Autodesk Fusion 360 part; units mm, degrees
note: some values were not read from the file. Chosen so that the rebuilt part matches the saved one: which bodies a step acts on; which face or edge a step refers to. Set by a fixed rule: which sketch regions a step uses.
(part 2 of 2)
chamfer "Chamfer1" distance 0.1 angle 45 2 edges at (2.2467, -480.7059, 0) (382.2081, -629.6946, 0) on bodies 3 in component "Side_Panel"
sketch "Sketch1 (2)" plane through (0, 0, 0) normal (0, 0, 1) x (-1, 0, 0) in component "Side_Panel"
  circle A0 centre (-385.0517, 697.8099) radius 3.15
  circle A1 centre (-364.1017, 475.8227) radius 3.15
  circle A2 centre (-226.7218, 475.8227) radius 3.15
  circle A3 centre (-108.0319, 475.8227) radius 3.15
  circle A4 centre (29.3479, 475.8227) radius 3.15
  circle A5 centre (118.9878, 496.7727) radius 3.15
  circle A6 centre (118.9878, 630.7975) radius 3.15
  circle A7 centre (118.9878, 697.8099) radius 3.15
  circle A8 centre (118.9878, 563.7851) radius 3.15
  circle A9 centre (98.0378, 475.8227) radius 3.15
  circle A10 centre (-39.342, 475.8227) radius 3.15
  circle A11 centre (-158.0319, 475.8227) radius 3.15
  circle A12 centre (-295.4117, 475.8227) radius 3.15
  circle A13 centre (-385.0517, 496.7727) radius 3.15
  circle A14 centre (-385.0517, 563.7851) radius 3.15
  arc A15 (-5.547, 484.7727) -> (-4.447, 484.7727) centre (-4.997, 481.7727) ccw
  line L0 (-5.547, 484.7727) -> (-82.4819, 484.7727)
  arc A16 (-83.5819, 484.7727) -> (-82.4819, 484.7727) centre (-83.0319, 481.7727) ccw
  line L1 (-83.5819, 484.7727) -> (-182.4819, 484.7727)
  arc A17 (-183.5819, 484.7727) -> (-182.4819, 484.7727) centre (-183.0319, 481.7727) ccw
  line L2 (-183.5819, 484.7727) -> (-260.5168, 484.7727)
  arc A18 (-261.6168, 484.7727) -> (-260.5168, 484.7727) centre (-261.0668, 481.7727) ccw
  line L3 (-261.6168, 484.7727) -> (-338.5517, 484.7727)
  arc A19 (-339.6517, 484.7727) -> (-338.5517, 484.7727) centre (-339.1017, 481.7727) ccw
  line L4 (-339.6517, 484.7727) -> (-376.1017, 484.7727)
  line L5 (-376.1017, 484.7727) -> (-376.1017, 521.2227)
  arc A20 (-376.1017, 522.3227) -> (-376.1017, 521.2227) centre (-379.1017, 521.7727) ccw
  line L6 (-376.1017, 522.3227) -> (-376.1017, 596.7413)
  arc A21 (-376.1017, 597.8413) -> (-376.1017, 596.7413) centre (-379.1017, 597.2913) ccw
  line L7 (-376.1017, 597.8413) -> (-376.1017, 672.2599)
  arc A22 (-376.1017, 673.3599) -> (-376.1017, 672.2599) centre (-379.1017, 672.8099) ccw
  line L8 (-376.1017, 673.3599) -> (-376.1017, 722.8099)
  line L9 (-376.1017, 722.8099) -> (-387.1017, 722.8099)
  line L10 (-387.1017, 722.8099) -> (-387.1017, 702.8099)
  arc A23 (-389.1017, 700.8099) -> (-387.1017, 702.8099) centre (-389.1017, 702.8099) ccw
  line L11 (-389.1017, 700.8099) -> (-389.1017, 473.7727)
  arc A24 (-389.1017, 473.7727) -> (-387.1017, 471.7727) centre (-387.1017, 473.7727) ccw
  line L12 (-387.1017, 471.7727) -> (-155.0319, 471.7727)
  arc A25 (-153.0319, 473.7727) -> (-155.0319, 471.7727) centre (-153.0319, 471.7727) ccw
  line L13 (-153.0319, 473.7727) -> (-113.0319, 473.7727)
  arc A26 (-111.0319, 471.7727) -> (-113.0319, 473.7727) centre (-113.0319, 471.7727) ccw
  line L14 (-111.0319, 471.7727) -> (121.0378, 471.7727)
  arc A27 (121.0378, 471.7727) -> (123.0378, 473.7727) centre (121.0378, 473.7727) ccw
  line L15 (123.0378, 473.7727) -> (123.0378, 700.8099)
  arc A28 (121.0378, 702.8099) -> (123.0378, 700.8099) centre (123.0378, 702.8099) ccw
  line L16 (121.0378, 702.8099) -> (121.0378, 722.8099)
  line L17 (121.0378, 722.8099) -> (110.0378, 722.8099)
  line L18 (110.0378, 722.8099) -> (110.0378, 673.3599)
  arc A29 (110.0378, 672.2599) -> (110.0378, 673.3599) centre (113.0378, 672.8099) ccw
  line L19 (110.0378, 672.2599) -> (110.0378, 597.8413)
  arc A30 (110.0378, 596.7413) -> (110.0378, 597.8413) centre (113.0378, 597.2913) ccw
  line L20 (110.0378, 596.7413) -> (110.0378, 522.3227)
  arc A31 (110.0378, 521.2227) -> (110.0378, 522.3227) centre (113.0378, 521.7727) ccw
  line L21 (110.0378, 521.2227) -> (110.0378, 484.7727)
  line L22 (110.0378, 484.7727) -> (73.5878, 484.7727)
  arc A32 (72.4878, 484.7727) -> (73.5878, 484.7727) centre (73.0378, 481.7727) ccw
  line L23 (72.4878, 484.7727) -> (-4.447, 484.7727)
  circle A33 centre (-385.0517, 630.7975) radius 3.15
  line L24 (-133.0319, 473.7727) -> (-133.0319, 484.7727)
  constraint midpoint L13 L24.start
  constraint midpoint L1 L24.end
split "Split1'" by curves path "Sketch1 (2)" along L24 bodies 3 makes body 4 at (-115.4304, -706.7068, -4) in component "Side_Panel"
chamfer "Chamfer2'" distance 0.4 angle 45 2 faces at (-115.4304, -706.7068, -4) (381.6101, -706.6822, -4) on bodies 3 4 in component "Side_Panel"
extrude "Extrude17" add sketch "Master Sketch" against normal blind 5 separate body contours L21 L24 L27 L28 A72 L41 L42 A150 | L22 A53 L24 L27 L28 L29 L32 A62 A63 L35 L36 A72 A150 | L21 L28 L39 L41 L42 | L27 A150 | L27 A150 | A53 L29 L32 L35 | L21 L25 L28 L39 L40 L41 | L21 L24 L25 L28 L30 A73 L40 L41 A151 | L22 L23 A52 L24 L25 L26 L28 L30 A67 A68 L37 A73 A151 | L25 L26 A67 L37 | L30 A151 | L30 A151 | L22 L23 A52 L28 | L22 L28 A62 L36 | A50 | A51 | A54 | A55 | A56 | A57 | A58 | A59 | A60 | A61 | A64 | A65 | A66 | A69 | A70 | A71 makes body 5 in component "Top_Panel"
extrude "Extrude18" cut sketch "Master Sketch" against normal blind 90 contours L21 L28 L39 L41 L42 | L21 L25 L28 L39 L40 L41 bodies 5 in component "Top_Panel"
extrude "Extrude19" cut sketch "Master Sketch" against normal blind 3.1 contours A50 | A51 | A54 | A55 | A56 | A57 | A58 | A59 | A60 | A61 | A64 | A65 | A66 | A69 | A70 | A71 bodies 5 in component "Top_Panel"
extrude "Extrude20" cut sketch "Master Sketch" against normal blind 3.75 contours L21 L24 L27 L28 A72 L41 L42 A150 | L21 L24 L25 L28 L30 A73 L40 L41 A151 bodies 5 in component "Top_Panel"
revolve "Revolve10" cut sketch "Master Sketch" angle 360 about axis through (801.9622, -187.8424, 0) along (0, 1, 0) contours A53 L29 L32 L35 bodies 5 in component "Top_Panel"
revolve "Revolve11" cut sketch "Master Sketch" angle 360 about axis through (803.9622, 68.2273, 0) along (1, 0, 0) contours L22 L23 A52 L28 | L22 L28 A62 L36 bodies 5 in component "Top_Panel"
revolve "Revolve12" cut sketch "Master Sketch" angle 360 about axis through (1314.1017, 66.2273, 0) along (0, -1, 0) contours L25 L26 A67 L37 bodies 5 in component "Top_Panel"
chamfer "Chamfer7" distance 1 angle 45 1 faces at (979.342, 61.5607, -5) on bodies 5 in component "Top_Panel"
sketch "Sketch3" plane through (0, 0, 0) normal (0, 0, 1) x (-1, 0, 0) in component "Top_Panel"
  arc A0 (-1314.1017, 165.8424) -> (-1312.1017, 167.8424) centre (-1314.1017, 167.8424) ccw
  line L0 (-1314.1017, 165.8424) -> (-1314.1017, -66.2273)
  arc A1 (-1314.1017, -66.2273) -> (-1312.1017, -68.2273) centre (-1312.1017, -66.2273) ccw
  line L1 (-1312.1017, -68.2273) -> (-1080.0319, -68.2273)
  arc A2 (-1078.0319, -66.2273) -> (-1080.0319, -68.2273) centre (-1078.0319, -68.2273) ccw
  line L2 (-1078.0319, -66.2273) -> (-1038.0319, -66.2273)
  arc A3 (-1036.0319, -68.2273) -> (-1038.0319, -66.2273) centre (-1038.0319, -68.2273) ccw
  line L3 (-1036.0319, -68.2273) -> (-803.9622, -68.2273)
  arc A4 (-803.9622, -68.2273) -> (-801.9622, -66.2273) centre (-803.9622, -66.2273) ccw
  line L4 (-801.9622, -66.2273) -> (-801.9622, 165.8424)
  arc A5 (-803.9622, 167.8424) -> (-801.9622, 165.8424) centre (-801.9622, 167.8424) ccw
  line L5 (-803.9622, 167.8424) -> (-803.9622, 187.8424)
  line L6 (-803.9622, 187.8424) -> (-813.9622, 187.8424)
  line L7 (-813.9622, 187.8424) -> (-813.9622, 104.6563)
  arc A6 (-813.9622, 104.6563) -> (-813.9622, 101.0286) centre (-811.9622, 102.8424) ccw
  line L8 (-813.9622, 101.0286) -> (-813.9622, -55.2273)
  arc A7 (-814.9622, -56.2273) -> (-813.9622, -55.2273) centre (-814.9622, -55.2273) ccw
  line L9 (-814.9622, -56.2273) -> (-1301.1017, -56.2273)
  arc A8 (-1302.1017, -55.2273) -> (-1301.1017, -56.2273) centre (-1301.1017, -55.2273) ccw
  line L10 (-1302.1017, -55.2273) -> (-1302.1017, 101.0286)
  arc A9 (-1302.1017, 101.0286) -> (-1302.1017, 104.6563) centre (-1304.1017, 102.8424) ccw
  line L11 (-1302.1017, 104.6563) -> (-1302.1017, 187.8424)
  line L12 (-1302.1017, 187.8424) -> (-1312.1017, 187.8424)
  line L13 (-1312.1017, 187.8424) -> (-1312.1017, 167.8424)
  circle A10 centre (-1310.0517, 162.8424) radius 3.05
  circle A11 centre (-1289.1017, -64.1773) radius 3.05
  circle A12 centre (-1033.0319, -64.1773) radius 3.05
  circle A13 centre (-806.0122, -43.2273) radius 3.05
  circle A14 centre (-806.0122, 162.8424) radius 3.05
  circle A15 centre (-826.9622, -64.1773) radius 3.05
  circle A16 centre (-1083.0319, -64.1773) radius 3.05
  circle A17 centre (-1310.0517, -43.2273) radius 3.05
  circle A18 centre (-1310.0517, 94.1525) radius 3.05
  circle A19 centre (-1220.4117, -64.1773) radius 3.05
  circle A20 centre (-964.342, -64.1773) radius 3.05
  circle A21 centre (-806.0122, 25.4626) radius 3.05
  circle A22 centre (-806.0122, 94.1525) radius 3.05
  circle A23 centre (-895.6521, -64.1773) radius 3.05
  circle A24 centre (-1151.7218, -64.1773) radius 3.05
  circle A25 centre (-1310.0517, 25.4626) radius 3.05
  line L14 (-1058.0319, -66.2273) -> (-1058.0319, -56.2273)
  constraint midpoint L2 L14.start
  constraint midpoint L9 L14.end
split "Split3" by curves path "Sketch3" along L14 bodies 5 makes body 6 at (894.3187, 61.2273, -5) in component "Top_Panel"
copy_body "CopyPasteBodies2" bodies 6 5 2 1 makes body 7 makes body 8 makes body 9 makes body 10 in component "Top_Panel_with_Handle"
extrude "Extrude3'" cut sketch "Master Sketch" against normal blind 80 contours L27 A150 | L27 A150 | L30 A151 | L30 A151 | A148 | A149 bodies 7 8 9 10 in component "Top_Panel_with_Handle"
extrude "Extrude9'" add sketch "Master Sketch" against normal blind 5 separate body contours L72 A124 L75 L76 L78 L84 L85 L87 L100 | L72 L76 L79 L86 A141 L101 | L72 L86 L99 L100 L101 | L74 L75 L76 L84 L85 L87 | L76 L79 L86 A141 | L72 A124 A125 L77 L78 L85 L86 A142 L93 L99 | L74 L75 L85 L87 L88 | L75 L78 L82 L85 L87 L88 A146 L96 | L73 L81 L82 A135 L89 L97 | L73 L77 L78 A128 L82 L85 A143 L92 A146 L95 | L73 L81 A135 L89 | L73 L82 L95 L96 L97 L98 | L77 A128 L85 L92 | L77 L85 A142 L93 | A126 | A127 | A129 | A130 | A131 | A132 | A133 | A134 | A136 | A137 | A138 | A139 | A140 | A144 | A145 | A147 makes body 11 in component "Side_Panel"
extrude "Extrude10'" cut sketch "Master Sketch" against normal blind 60 contours L74 L75 L76 L84 L85 L87 | L74 L75 L85 L87 L88 bodies 11 in component "Side_Panel"
extrude "Extrude11" cut sketch "Master Sketch" against normal blind 3.1 contours A126 | A127 | A129 | A130 | A131 | A132 | A133 | A134 | A136 | A137 | A138 | A139 | A140 | A144 | A145 | A147 bodies 11 in component "Side_Panel"
revolve "Revolve7" cut sketch "Master Sketch" angle 360 about axis through (801.9622, -732.8099, 0) along (0, 1, 0) contours L73 L81 A135 L89 bodies 11 in component "Side_Panel"
revolve "Revolve8" cut sketch "Master Sketch" angle 360 about axis through (803.9622, -481.7727, 0) along (1, 0, 0) contours L77 A128 L85 L92 | L77 L85 A142 L93 bodies 11 in component "Side_Panel"
extrude "Extrude12" cut sketch "Master Sketch" against normal blind 3.75 contours L72 A124 L75 L76 L78 L84 L85 L87 L100 | L75 L78 L82 L85 L87 L88 A146 L96 bodies 11 in component "Side_Panel"
revolve "Revolve9" cut sketch "Master Sketch" angle 360 about axis through (1314.1017, -483.7727, 0) along (0, -1, 0) contours L76 L79 L86 A141 bodies 11 in component "Side_Panel"
sketch "Sketch3 (2)" plane through (0, 0, 0) normal (0, 0, 1) x (-1, 0, 0) in component "Side_Panel"
  arc A0 (-1314.1017, 710.8099) -> (-1312.1017, 712.8099) centre (-1314.1017, 712.8099) ccw
  line L0 (-1314.1017, 710.8099) -> (-1314.1017, 483.7727)
  arc A1 (-1314.1017, 483.7727) -> (-1312.1017, 481.7727) centre (-1312.1017, 483.7727) ccw
  line L1 (-1312.1017, 481.7727) -> (-1080.0319, 481.7727)
  arc A2 (-1078.0319, 483.7727) -> (-1080.0319, 481.7727) centre (-1078.0319, 481.7727) ccw
  line L2 (-1078.0319, 483.7727) -> (-1038.0319, 483.7727)
  arc A3 (-1036.0319, 481.7727) -> (-1038.0319, 483.7727) centre (-1038.0319, 481.7727) ccw
  line L3 (-1036.0319, 481.7727) -> (-803.9622, 481.7727)
  arc A4 (-803.9622, 481.7727) -> (-801.9622, 483.7727) centre (-803.9622, 483.7727) ccw
  line L4 (-801.9622, 483.7727) -> (-801.9622, 710.8099)
  arc A5 (-803.9622, 712.8099) -> (-801.9622, 710.8099) centre (-801.9622, 712.8099) ccw
  line L5 (-803.9622, 712.8099) -> (-803.9622, 732.8099)
  line L6 (-803.9622, 732.8099) -> (-813.9622, 732.8099)
  line L7 (-813.9622, 732.8099) -> (-813.9622, 494.7727)
  arc A6 (-814.9622, 493.7727) -> (-813.9622, 494.7727) centre (-814.9622, 494.7727) ccw
  line L8 (-814.9622, 493.7727) -> (-1301.1017, 493.7727)
  arc A7 (-1302.1017, 494.7727) -> (-1301.1017, 493.7727) centre (-1301.1017, 494.7727) ccw
  line L9 (-1302.1017, 494.7727) -> (-1302.1017, 732.8099)
  line L10 (-1302.1017, 732.8099) -> (-1312.1017, 732.8099)
  line L11 (-1312.1017, 732.8099) -> (-1312.1017, 712.8099)
  circle A8 centre (-1310.0517, 707.8099) radius 3.05
  circle A9 centre (-1289.1017, 485.8227) radius 3.05
  circle A10 centre (-1033.0319, 485.8227) radius 3.05
  circle A11 centre (-806.0122, 573.7851) radius 3.05
  circle A12 centre (-806.0122, 640.7975) radius 3.05
  circle A13 centre (-964.342, 485.8227) radius 3.05
  circle A14 centre (-1220.4117, 485.8227) radius 3.05
  circle A15 centre (-1310.0517, 640.7975) radius 3.05
  circle A16 centre (-1310.0517, 506.7727) radius 3.05
  circle A17 centre (-1083.0319, 485.8227) radius 3.05
  circle A18 centre (-806.0122, 506.7727) radius 3.05
  circle A19 centre (-806.0122, 707.8099) radius 3.05
  circle A20 centre (-895.6521, 485.8227) radius 3.05
  circle A21 centre (-1151.7218, 485.8227) radius 3.05
  circle A22 centre (-1310.0517, 573.7851) radius 3.05
  line L12 (-1058.0319, 483.7727) -> (-1058.0319, 493.7727)
  circle A23 centre (-826.9622, 485.8227) radius 3.05
  constraint midpoint L2 L12.start
  constraint midpoint L8 L12.end
chamfer "Chamfer5" distance 0.1 angle 45 15 edges at (803.1686, -706.707, 0) (803.1686, -639.6946, 0) (803.1686, -572.6822, 0) (803.1686, -505.6697, 0) (892.8085, -484.7197, 0) (961.4984, -484.7197, 0) (1030.1883, -484.7197, 0) (1080.1883, -484.7197, 0) (1148.8782, -484.7197, 0) (1217.5681, -484.7197, 0) (1307.2081, -505.6697, 0) (1286.2581, -484.7197, 0) (1307.2081, -572.6822, 0) (1307.2081, -639.6946, 0) (1307.2081, -706.707, 0) on bodies 11 in component "Side_Panel"
chamfer "Chamfer5" distance 0.1 angle 45 1 edges at (824.1186, -484.7197, 0) on bodies 11 in component "Side_Panel"
chamfer "Chamfer6" distance 1 angle 45 1 faces at (979.342, -488.4393, -5) on bodies 11 in component "Side_Panel"
split "Split4" by curves path "Sketch3 (2)" along L12 bodies 11 makes body 12 at (894.3187, -488.7727, -5) in component "Side_Panel"
copy_body "CopyPasteBodies2'" bodies 3 11 4 12 makes body 13 makes body 14 makes body 15 makes body 16 in component "Side_Panel_With_270_Hinge"
extrude "Extrude4'" cut sketch "Master Sketch" against normal blind 55 contours L54 L69 L70 L71 | L48 L65 L66 L67 L68 | A74 | A117 | L72 L86 L99 L100 L101 | L73 L82 L95 L96 L97 L98 | A129 | A137 bodies 13 14 15 16 in component "Side_Panel_With_270_Hinge"
copy_body "CopyPasteBodies3" bodies 3 11 4 12 makes body 17 makes body 18 makes body 19 makes body 20 in component "Side_Panel_With_270_Hinge"
extrude "Extrude5" add 1 faces at (898.3187, -496.4393, -3.75) along direction (0, 0, 1) blind 1 on bodies 20 bodies 20 18 in component "Side_Panel_With_270_Hinge"
extrude "Extrude21" cut sketch "Master Sketch" against normal blind 3.75 contours L27 A150 picked at (814.1857, -102.9745) bodies 6 in component "Top_Panel"
extrude "Extrude22" cut sketch "Master Sketch" against normal blind 3.75 contours L30 A151 picked at (1301.9548, -102.4575) bodies 5 in component "Top_Panel"
extrude "Extrude6" cut 1 faces at (898.3187, -496.4393, -2.75) along direction (0, 0, -1) blind 1 on bodies 20 bodies 20 in component "Side_Panel_With_270_Hinge"
split "Split1''" by curves path "Sketch3 (2)" along L12 bodies 20 makes body 21 at (894.3187, -488.7727, -5) in component "Side_Panel_With_270_Hinge"
component "Top_Panel" placed x (1, 0, 0) y (0, 1, 0) z (0, 0, 1) at (0, 0, 0)
component "Top_Panel_with_Handle" placed x (1, 0, 0) y (0, 1, 0) z (0, 0, 1) at (0, 0, 0)
component "Side_Panel" placed x (1, 0, 0) y (0, 1, 0) z (0, 0, 1) at (0, 0, 0)
component "Side_Panel_With_270_Hinge" placed x (1, 0, 0) y (0, 1, 0) z (0, 0, 1) at (0, 0, 0)
equation "BaseTopPanelWidth = 483 mm"
equation "BaseTopPanelHeight = 483 mm"
equation "TopPanelWidth = BaseTopPanelWidth * 1.0065"
equation "TopPanelHeight = BaseTopPanelHeight * 1.0065"
equation "MagnetWidth = 6.1 mm"
equation "MagnetDepth = 3.1 mm"
equation "ScrewHoleDiameter = 3.4 mm"
equation "ScrewWidth = 5.9 mm"
equation "ScrewInset = 50 mm"
equation "d15 = MagnetWidth"
equation "d21 = ScrewInset / 2"
equation "FrameWidth = TopPanelWidth + 26 mm"
equation "d25 = ScrewHoleDiameter"
equation "d26 = ScrewWidth"
equation "d27 = ScrewHoleDiameter"
equation "d28 = ScrewWidth"
equation "d31 = ScrewHoleDiameter"
equation "d32 = ScrewWidth"
equation "d34 = ScrewInset"
equation "d35 = ScrewInset"
equation "FrameDepth = TopPanelHeight + 26 mm"
equation "d46 = MagnetWidth"
equation "d47 = ScrewHoleDiameter"
equation "d48 = ScrewWidth"
equation "d49 = MagnetWidth"
equation "d57 = ScrewInset / 2"
equation "d58 = ScrewHoleDiameter"
equation "d59 = ScrewWidth"
equation "d60 = ScrewHoleDiameter"
equation "d61 = ScrewWidth"
equation "d62 = ScrewHoleDiameter"
equation "d63 = ScrewWidth"
equation "d64 = ScrewInset"
equation "d66 = ScrewInset"
equation "d67 = FrameDepth / 2"
equation "d68 = FrameWidth"
equation "ScrewDepth = 3.1 mm"
equation "d337 = MagnetWidth"
equation "d338 = ScrewInset / 2 + ( FrameWidth / 2 - ScrewInset ) / 3"
equation "d339 = MagnetWidth"
equation "d340 = ScrewInset / 2 + ( FrameWidth / 2 - ScrewInset ) / 3"
equation "d341 = MagnetWidth"
equation "d342 = MagnetWidth"
equation "d343 = ScrewInset / 2"
equation "d344 = MagnetWidth"
equation "d346 = MagnetWidth"
equation "d348 = MagnetWidth"
equation "d350 = ScrewInset / 2 + ( FrameDepth / 2 - ScrewInset ) / 3"
equation "d351 = ScrewInset / 2 + ( FrameDepth / 2 - ScrewInset ) / 3"
equation "d352 = ScrewInset / 2"
equation "d358 = MagnetWidth"
equation "d360 = ScrewInset / 2"
equation "d377 = MagnetWidth"
equation "d379 = ScrewInset / 2"
equation "d389 = FrameDepth / 2"
equation "d390 = FrameWidth"
equation "d393 = MagnetWidth"
equation "d394 = ScrewInset / 2 + ( FrameWidth / 2 - ScrewInset ) / 3"
equation "d395 = MagnetWidth"
equation "d396 = ScrewInset / 2 + ( FrameWidth / 2 - ScrewInset ) / 3"
equation "d398 = MagnetWidth"
equation "d399 = ScrewInset / 2"
equation "d400 = MagnetWidth"
equation "d401 = MagnetWidth"
equation "d402 = MagnetWidth"
equation "d403 = ScrewInset / 2 + ( FrameWidth / 2 - ScrewInset ) / 3"
equation "d404 = ScrewInset / 2 + ( FrameWidth / 2 - ScrewInset ) / 3"
equation "d405 = ScrewInset / 2"
equation "d417 = MagnetWidth"
equation "d419 = ScrewInset / 2"
equation "d420 = ScrewHoleDiameter"
equation "d421 = ScrewWidth"
equation "d422 = ScrewHoleDiameter"
equation "d423 = ScrewWidth"
equation "d424 = ScrewHoleDiameter"
equation "d425 = ScrewWidth"
equation "d427 = ScrewInset"
equation "d428 = ScrewInset"
equation "d433 = MagnetWidth"
equation "d434 = ScrewHoleDiameter"
equation "d435 = ScrewWidth"
equation "d436 = MagnetWidth"
equation "d438 = ScrewInset / 2"
equation "d439 = ScrewHoleDiameter"
equation "d440 = ScrewWidth"
equation "d441 = ScrewHoleDiameter"
equation "d442 = ScrewWidth"
equation "d443 = ScrewHoleDiameter"
equation "d444 = ScrewWidth"
equation "d445 = ScrewInset"
equation "d447 = ScrewInset"
equation "d448 = FrameHeight / 2"
equation "d449 = FrameWidth"
equation "d452 = MagnetWidth"
equation "d453 = ScrewInset / 2 + ( FrameWidth / 2 - ScrewInset ) / 3"
equation "d454 = MagnetWidth"
equation "d455 = ScrewInset / 2 + ( FrameWidth / 2 - ScrewInset ) / 3"
equation "d456 = MagnetWidth"
equation "d457 = MagnetWidth"
equation "d458 = ScrewInset / 2"
equation "d459 = MagnetWidth"
equation "d460 = MagnetWidth"
equation "d461 = MagnetWidth"
equation "d462 = ScrewInset / 2 + ( FrameHeight / 2 - ScrewInset ) / 3"
equation "d463 = ScrewInset / 2 + ( FrameHeight / 2 - ScrewInset ) / 3"
equation "d464 = ScrewInset / 2"
equation "d472 = MagnetWidth"
equation "d474 = ScrewInset / 2"
equation "d488 = MagnetWidth"
equation "d490 = ScrewInset / 2"
equation "d500 = FrameHeight / 2"
equation "d501 = FrameWidth"
equation "d504 = MagnetWidth"
equation "d505 = ScrewInset / 2 + ( FrameWidth / 2 - ScrewInset ) / 3"
equation "d506 = MagnetWidth"
equation "d507 = ScrewInset / 2 + ( FrameWidth / 2 - ScrewInset ) / 3"
equation "d508 = MagnetWidth"
equation "d509 = ScrewInset / 2"
equation "d510 = MagnetWidth"
equation "d511 = MagnetWidth"
equation "d512 = MagnetWidth"
equation "d513 = ScrewInset / 2 + ( FrameHeight / 2 - ScrewInset ) / 3"
equation "d514 = ScrewInset / 2 + ( FrameHeight / 2 - ScrewInset ) / 3"
equation "d515 = ScrewInset / 2"
equation "d532 = -ScrewDepth"
equation "d534 = -MagnetDepth"
equation "d541 = ( 170 / 2 ) * 1 mm"
equation "d543 = ( 170 / 2 ) * 1 mm"
equation "PanelDepth = 3 mm"
equation "FoamDepth = 3 mm"
equation "PanelSquish = 0.25 mm"
equation "PanelGlassLedgeDepth = PanelDepth + FoamDepth - 2 mm - PanelSquish"
equation "BaseSidePanelHeight = 473 mm"
equation "SidePanelHeight = BaseSidePanelHeight * 1.0065"
equation "FrameHeight = SidePanelHeight + 26 mm"
equation "d582 = -ScrewDepth"
equation "d584 = -MagnetDepth"
equation "d615 = -MagnetDepth"
equation "d617 = -PanelGlassLedgeDepth"
equation "d629 = -MagnetDepth"
equation "d633 = -PanelGlassLedgeDepth"
named bodies: "Top_Right_and_Bottom_Left_x2", "Top_Left_and_Bottom_Right_x2", "Panel_Top_Right_and_Bottom_Left_x2", "Panel_Top_Left_and_Bottom_Right_x2", "Hinge_Top_Right_and_Bottom_Left_x1", "Hinge_Panel_Top_Right_and_Bottom_Left_x1", "Hinge_Top_Left_and_Bottom_Right_x1", "Hinge_Panel_Top_Left_and_Bottom_Right_x1", "Top_Right_and_Bottom_Left_x2 (1)", "Panel_Top_Right_and_Bottom_Left_x2 (1)", "Top_Left_and_Bottom_Right_x2 (1)", "Panel_Top_Left_and_Bottom_Right_x2 (1)", "Top_Right_and_Bottom_Left_x1", "Panel_Top_Right_and_Bottom_Left_x1", "Top_Left_and_Bottom_Right_x1", "Panel_Top_Left_and_Bottom_Right_x1"
